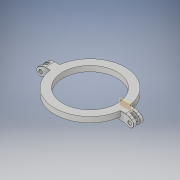
# Autodesk Inventor part: aret-ring
Saved by Autodesk Inventor 2019 (Build 230136000, 136)
## iProperties
Created: 2022-10-05
Part Number: aret-ring
Material: Generic
Document SubType Name: Modeling
Designer: Karbosch
Mass: 22.9453 g
Surface Area: 93.8239 cm^2
Volume: 22.9453 cm^3
Density: 1 g/cm^3
Appearance: Default
Author: Karbosch
Autodesk Inventor part; units mm, degrees
ref_plane "YZ Plane" through (0, 0, 0) normal (1, 0, 0) x (0, 1, 0)
ref_plane "XZ Plane" through (0, 0, 0) normal (0, 1, 0) x (-1, 0, 0)
ref_plane "XY Plane" through (0, 0, 0) normal (0, 0, 1) x (1, 0, 0)
sketch "Sketch153" plane through (0, 0, 0) normal (1, 0, 0) x (0, 1, 0)
  line L0 (0, 0) -> (10, 0)
  line L1 (10, 0) -> (10, -15)
  line L2 (10, -15) -> (0, -15)
  line L3 (0, -15) -> (0, 0)
  line L4 (0, 0) -> (0, 50)
  line L5 (0, 50) -> (25, 50)
  dimension "d741" = 10
  dimension "d742" = 15
  dimension "d743" = 50
  constraints: 12 end point, 2 horizontal, 2 parallel, 1 perpendicular, 1 vertical
  measures "d741" distance of L1.end L2.end
  measures "d742" distance of L0.end L1.end
  measures "d743" distance of L0.start L4.end
revolve "Revolution11" add sketch "Sketch153" angle 180 about axis through (0, 0, 50) along (0, -1, 0)
ref_plane "Work Plane62" through (65, 10, 50) normal (0, 0, 1) x (1, 0, 0)
sketch "Sketch154" plane through (65, 10, 50) normal (0, 0, 1) x (1, 0, 0)
  line L0 (0, -10) -> (15, -10) construction
  arc A0 (12.9904, -17.5) -> (20.4904, -4.5096) centre (16.7404, -11.0048) ccw
  line L1 (20.4904, -4.5096) -> (16.1603, -2.0096)
  line L2 (20.4904, -4.5096) -> (25.4904, -4.5096) construction
  arc A1 (16.1603, -2.0096) -> (8.6603, 0) centre (8.6603, -15) ccw
  line L3 (-65, 0) -> (0, 0) projected
  line L4 (8.6603, 0) -> (0, 0)
  arc A2 (12.9904, -17.5) -> (5.4904, -15.4904) centre (5.4904, -30.4904) ccw
  line L5 (-65, -10) -> (-15, -10) projected
  arc A3 (-15, -10) -> (5.4904, -15.4904) centre (5.4904, 25.4904) ccw
  line L6 (0, 0) -> (-15, 0)
  line L7 (-15, -10) -> (-15, 0)
  line L8 (-15, -10) -> (-15, 0) projected
  circle A4 centre (16.7404, -11.0048) radius 3.15
  dimension "d745" = 15
  dimension "d747" = 7.5
  dimension "d748" = 5
  dimension "d749" = 150
  dimension "d750" = 15
  dimension "d751" = 15
  dimension "d752" = 6.3
  constraints: 12 end point, 8 point on circle, 5 centre point, 3 horizontal, 3 tangent, 1 coincident, 1 collinear, 1 equal length, 1 point on line
  measures "d745" distance of L0.start A0.start
  measures "d747" radius of A0
  measures "d748" distance of L1.start L1.end
  measures "d749" angle of L2 L1
  measures "d750" radius of A1
  measures "d751" radius of A2
  measures "d752" diameter of A4
extrude "Extrusion114" add sketch "Sketch154" along normal mid plane 17.9
sketch "Sketch155" plane through (65, 10, 50) normal (0, 0, 1) x (1, 0, 0)
  arc A0 (12.9904, -17.5) -> (20.4904, -4.5096) centre (16.7404, -11.0048) ccw projected
  circle A1 centre (16.7404, -11.0048) radius 3.15 projected
  arc A2 (13.8257, -0.9175) -> (7.2992, -15.5998) centre (16.7404, -11.0048) ccw
  line L0 (-15, -10) -> (-0.6191, -10) projected
  arc A3 (-15, -10) -> (5.4904, -15.4904) centre (5.4904, 25.4904) ccw projected
  arc A4 (12.9904, -17.5) -> (5.4904, -15.4904) centre (5.4904, -30.4904) ccw projected
  arc A5 (12.9904, -17.5) -> (20.4904, -4.5096) centre (16.7404, -11.0048) ccw projected
  line L1 (20.4904, -4.5096) -> (16.1603, -2.0096) projected
  arc A6 (16.1603, -2.0096) -> (8.6603, 0) centre (8.6603, -15) ccw projected
  line L2 (8.6603, 0) -> (-0.6191, 0) projected
  line L3 (-0.6191, -10) -> (-0.6191, 0) projected
  circle A7 centre (16.7404, -11.0048) radius 3.15 projected
  point P0 (-65, -10)
  dimension "d755" = 21
  constraints: 4 point on circle, 1 centre point, 1 coincident
  measures "d755" diameter of A2
extrude "Extrusion115" cut sketch "Sketch155" along normal mid plane 6.1 contours A4 A2 A6 L1 A0
fillet "Fillet10" radius 1 2 edges at (78.8257, 9.0825, 50) (72.2992, -5.5998, 50)
fillet "Fillet11" radius 0.4 28 edges at (77.4031, 9.5255, 53.05) (80.0165, 8.5867, 53.05) (88.2356, -4.7548, 53.05) (71.5329, -5.5267, 53.05) (75.2408, -6.2625, 53.05) (83.3253, 6.7404, 53.05) (69.0206, 10, 58.95) (83.3253, 6.7404, 58.95) (88.2356, -4.7548, 58.95) (74.3727, -6.0015, 58.95) (59.8838, -4.094, 58.95) (77.5425, 9.4889, 58.95) (88.2356, -4.7548, 46.95) (71.5329, -5.5267, 46.95) (75.2408, -6.2625, 46.95) (77.4031, 9.5255, 46.95) (80.0165, 8.5867, 46.95) (83.3253, 6.7404, 46.95) (88.2356, -4.7548, 41.05) (74.3727, -6.0015, 41.05) (59.8838, -4.094, 41.05) (77.5425, 9.4889, 41.05) (69.0206, 10, 41.05) (83.3253, 6.7404, 41.05) (78.5904, -1.0048, 41.05) (78.5904, -1.0048, 53.05) (78.5904, -1.0048, 46.95) (78.5904, -1.0048, 58.95)
mirror "Mirror1" about plane through (0, 5, -7.5) normal (-1, 0, 0)
body "Solid9"
